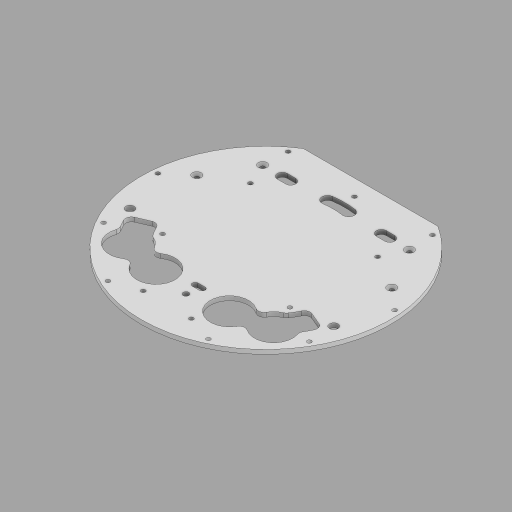
# Autodesk Inventor part: V_2
Saved by Autodesk Inventor 2024.2 (Build 282272000, 272)
## iProperties
Created: 2023-12-16
Part Number: V_2
Material: Типовые
Document SubType Name: Modeling
Designer: Фёдор
Density: 1 g/cm^3
Appearance: По умолчанию
Author: Фёдор
Autodesk Inventor part; units mm, degrees
ref_plane "YZ Plane" through (0, 0, 0) normal (1, 0, 0) x (0, 1, 0)
ref_plane "XZ Plane" through (0, 0, 0) normal (0, 1, 0) x (-1, 0, 0)
ref_plane "XY Plane" through (0, 0, 0) normal (0, 0, 1) x (1, 0, 0)
sketch "Эскиз1" plane through (0, 0, 0) normal (0, 1, 0) x (-1, 0, 0)
  arc A0 (110.5702, -95.2576) -> (50, 9.653) centre (25, -74.7211) ccw
  line L0 (102.2104, -90.4311) -> (110.5702, -95.2576) construction
  line L1 (102.2104, -90.4311) -> (77.2104, -133.7324) construction
  line L2 (85.5702, -138.5589) -> (77.2104, -133.7324) construction
  arc A1 (70, -150.3452) -> (85.5702, -138.5589) centre (25, -74.7211) ccw
  line L3 (-20, -150.3452) -> (70, -150.3452)
  arc A2 (-35.5702, -138.5589) -> (-20, -150.3452) centre (25, -74.7211) ccw
  line L4 (-27.2104, -133.7324) -> (-35.5702, -138.5589) construction
  line L5 (-27.2104, -133.7324) -> (-52.2104, -90.4311) construction
  line L6 (-60.5702, -95.2576) -> (-52.2104, -90.4311) construction
  arc A3 (0, 9.653) -> (-60.5702, -95.2576) centre (25, -74.7211) ccw
  line L7 (0, 0) -> (0, 9.653) construction
  line L8 (0, 0) -> (50, 0) construction
  line L9 (50, 9.653) -> (50, 0) construction
  line L10 (25, -74.7211) -> (25, 8.2789) construction
  line L11 (0, 0) -> (50, 0) construction
  line L12 (50, 0) -> (50, -10) construction
  line L13 (50, -10) -> (0, -10) construction
  line L14 (0, -10) -> (0, 0) construction
  line L15 (0, -5) -> (50, -5) construction
  circle A4 centre (8, -5) radius 1.5
  circle A5 centre (42, -5) radius 1.5
  circle A6 centre (93.8803, -94.8593) radius 1.5
  circle A7 centre (76.8803, -124.3042) radius 1.5
  circle A8 centre (-26.8803, -124.3042) radius 1.5
  circle A9 centre (-43.8803, -94.8593) radius 1.5
  circle A10 centre (25, -74.7211) radius 88
  point P0 (0, 0)
  point P1 (-35.5702, -138.5589)
  point P2 (85.5702, -138.5589)
  point P3 (110.5702, -95.2576)
  point P4 (50, 9.653)
  point P5 (0, 9.653)
  dimension "d25" = 50
  dimension "d26" = 10
  dimension "d27" = 3
  dimension "d28" = 3
  dimension "d29" = 8
  dimension "d30" = 8
  dimension "d33" = 360
  constraints: 32 end point, 10 centre point, 8 point on circle, 3 horizontal, 3 vertical, 2 coincident, 2 midpoint, 2 parallel, 2 point on line, 1 perpendicular, 45 other
  measures "d25" distance of L12.end L13.end
  measures "d26" distance of L11.end L12.end
  measures "d27" diameter of A4
  measures "d28" diameter of A5
  measures "d29" distance from line of L14 A4.centre
  measures "d30" distance from line of L12 A5.centre
extrude "Выдавливание1" add sketch "Эскиз1" along normal blind 3 contours A10 A1 L3 A2 A3 A0
sketch "Эскиз8" plane through (0, 3, 0) normal (0, 1, 0) x (1, 0, 0)
  circle A0 centre (-8, 5) radius 1.5 projected
  circle A1 centre (-42, 5) radius 1.5 projected
  circle A2 centre (-93.8803, 94.8593) radius 1.5 projected
  circle A3 centre (-76.8803, 124.3042) radius 1.5 projected
  circle A4 centre (26.8803, 124.3042) radius 1.5 projected
  circle A5 centre (43.8803, 94.8593) radius 1.5 projected
  arc A6 (-70, 150.3452) -> (20, 150.3452) centre (-25, 74.7211) ccw projected
  line L0 (-25, 74.7211) -> (-186.093, 74.7211) construction
  circle A7 centre (-25, 74.7211) radius 80
  line L1 (-25, 74.7211) -> (-112.6651, 82.3909) construction
  line L2 (-112.6651, 82.3909) -> (-108.6804, 82.0422) construction
  circle A8 centre (-108.6804, 82.0422) radius 1.5
  line L3 (-25, 74.7211) -> (-78.4735, 144.611) construction
  circle A9 centre (-76.0429, 141.4342) radius 1.5
  line L4 (-25, 74.7211) -> (-62.1904, -5.0339) construction
  line L5 (-25, 74.7211) -> (-101.2102, 30.7211) construction
  circle A10 centre (-60.4999, -1.4087) radius 1.5
  circle A11 centre (-97.7461, 32.7211) radius 1.5
  line L6 (-25, 74.7211) -> (-25, -13.2789) construction
  circle A12 centre (58.6804, 82.0422) radius 1.5
  circle A13 centre (26.0429, 141.4342) radius 1.5
  circle A14 centre (10.4999, -1.4087) radius 1.5
  circle A15 centre (47.7461, 32.7211) radius 1.5
  line L7 (-68, 140.8452) -> (18, 140.8452) projected
  line L8 (-25, 140.8452) -> (-25, 137.3452) construction
  circle A16 centre (-25, 137.3452) radius 1.5
  line L9 (20, 150.3452) -> (-70, 150.3452) projected
  point P0 (0, 0)
  dimension "d47" = 8
  dimension "d48" = 5
  dimension "d50" = 4
  dimension "d51" = 3
  dimension "d52" = 52.58
  dimension "d53" = 3
  dimension "d54" = 4
  dimension "d55" = 3
  dimension "d56" = 3
  dimension "d57" = 4
  dimension "d58" = 4
  dimension "d59" = 30
  dimension "d60" = 65
  dimension "d61" = 3.5
  dimension "d62" = 3
  constraints: 16 end point, 10 centre point, 5 point on circle, 4 point on line, 4 symmetric about line, 3 coincident, 2 horizontal, 1 midpoint, 1 vertical, 4 other
  measures "d47" radial gap between concentric circles of A6 A7
  measures "d48" angle of L1 L0
  measures "d50" distance of L1.end L2.end
  measures "d51" diameter of A8
  measures "d52" angle of L3 L0
  measures "d53" diameter of A9
  measures "d54" distance of L3.end A9.centre
  measures "d55" diameter of A10
  measures "d56" diameter of A11
  measures "d57" distance of L5.end A11.centre
  measures "d58" distance of L4.end A10.centre
  measures "d59" angle of L5 L0
  measures "d60" angle of L0 L4
  measures "d61" distance of L8.start L8.end
  measures "d62" diameter of A16
extrude "Выдавливание6" cut sketch "Эскиз8" against normal blind 10 contours A8 | A9 | A10 | A11 | A12 | A13 | A14 | A15 | A16
sketch "Эскиз10" plane through (0, 3, 0) normal (0, 1, 0) x (1, 0, 0)
  arc A0 (-70, 150.3452) -> (20, 150.3452) centre (-25, 74.7211) ccw projected
  line L0 (-72.591, 148.7421) -> (22.591, 148.7421)
  circle A1 centre (26.0429, 141.4342) radius 1.5 projected
  circle A2 centre (-60.4999, -1.4087) radius 1.5 projected
  circle A3 centre (-97.7461, 32.7211) radius 1.5 projected
  circle A4 centre (58.6804, 82.0422) radius 1.5 projected
  circle A5 centre (-25, 137.3452) radius 1.5 projected
  circle A6 centre (10.4999, -1.4087) radius 1.5 projected
  circle A7 centre (-108.6804, 82.0422) radius 1.5 projected
  circle A8 centre (47.7461, 32.7211) radius 1.5 projected
  circle A9 centre (-76.0429, 141.4342) radius 1.5 projected
  arc A10 (-70, 150.3452) -> (20, 150.3452) centre (-25, 74.7211) ccw projected
  line L1 (20, 150.3452) -> (-70, 150.3452) projected
  point P0 (0, 0)
  point P1 (20, 150.3452)
  dimension "d71" = 95.182
  constraints: 2 end point, 2 point on circle, 1 horizontal
  measures "d71" distance of L0.start L0.end
extrude "Выдавливание7" cut sketch "Эскиз10" against normal blind 10 contours L1 A0 L0
sketch "Эскиз11" plane through (0, 3, 0) normal (0, 1, 0) x (1, 0, 0)
  line L0 (22.591, 148.7421) -> (-72.591, 148.7421) projected
  arc A0 (-72.591, 148.7421) -> (22.591, 148.7421) centre (-25, 74.7211) ccw projected
  circle A1 centre (26.0429, 141.4342) radius 1.5 projected
  circle A2 centre (-60.4999, -1.4087) radius 1.5 projected
  circle A3 centre (-97.7461, 32.7211) radius 1.5 projected
  circle A4 centre (58.6804, 82.0422) radius 1.5 projected
  circle A5 centre (-25, 137.3452) radius 1.5 projected
  circle A6 centre (10.4999, -1.4087) radius 1.5 projected
  circle A7 centre (-108.6804, 82.0422) radius 1.5 projected
  circle A8 centre (47.7461, 32.7211) radius 1.5 projected
  circle A9 centre (-76.0429, 141.4342) radius 1.5 projected
  circle A10 centre (-25, 74.7211) radius 65
  line L1 (-74.6085, 116.7211) -> (24.6085, 116.7211)
  line L2 (22.591, 148.7421) -> (-72.591, 148.7421) projected
  line L3 (-80.3986, 108.7211) -> (30.3986, 108.7211) construction
  circle A11 centre (-70, 108.7211) radius 1.5
  circle A12 centre (20, 108.7211) radius 1.5
  circle A13 centre (-25, 74.7211) radius 56.5155 construction
  line L4 (-25, 74.7211) -> (-25, 9.7211) construction
  circle A14 centre (-25, 18.2056) radius 2
  line L5 (-74.0918, 46.7211) -> (24.0918, 46.7211) construction
  circle A15 centre (-70, 46.7211) radius 1.5
  circle A16 centre (20, 46.7211) radius 1.5
  point P0 (0, 0)
  dimension "d74" = 130
  dimension "d75" = 42
  dimension "d76" = 8
  dimension "d77" = 3
  dimension "d78" = 3
  dimension "d79" = 45
  dimension "d80" = 45
  dimension "d81" = 113.031
  dimension "d82" = 4
  dimension "d83" = 70
  dimension "d91" = 3
  dimension "d92" = 3
  dimension "d93" = 45
  dimension "d94" = 45
  dimension "d130" = 34
  dimension "d131" = 62
  dimension "d132" = 56.5155
  constraints: 8 end point, 8 point on circle, 7 centre point, 5 point on line, 3 horizontal, 2 coincident, 1 parallel, 1 vertical
  measures "d74" diameter of A10
  measures "d75" distance from line of L1 A0.centre
  measures "d76" distance between parallel lines of L1 L3
  measures "d77" diameter of A11
  measures "d78" diameter of A12
  measures "d79" horizontal distance of A11.centre A0.centre
  measures "d80" horizontal distance of A12.centre A0.centre
  measures "d81" diameter of A13
  measures "d82" diameter of A14
  measures "d83" distance between parallel lines of L1 L5
  measures "d91" diameter of A15
  measures "d92" diameter of A16
  measures "d93" horizontal distance of A0.centre A16.centre
  measures "d94" horizontal distance of A0.centre A15.centre
  measures "d130" distance from line of L3 A0.centre
  measures "d131" distance between parallel lines of L5 L3
  measures "d132" distance of A14.centre A0.centre
extrude "Выдавливание8" cut sketch "Эскиз11" against normal blind 10 contours A11 | A12 | A14 | A15 | A16
chamfer "Фаска3" [suppressed]
sketch "Эскиз12" plane through (0, 0, 0) normal (0, -1, 0) x (1, 0, 0)
  circle A0 centre (26.0429, -141.4342) radius 1.5 projected
  circle A1 centre (-60.4999, 1.4087) radius 1.5 projected
  circle A2 centre (-97.7461, -32.7211) radius 1.5 projected
  circle A3 centre (58.6804, -82.0422) radius 1.5 projected
  circle A4 centre (-25, -137.3452) radius 1.5 projected
  circle A5 centre (10.4999, 1.4087) radius 1.5 projected
  circle A6 centre (-108.6804, -82.0422) radius 1.5 projected
  circle A7 centre (47.7461, -32.7211) radius 1.5 projected
  circle A8 centre (-76.0429, -141.4342) radius 1.5 projected
  line L0 (-72.591, -148.7421) -> (22.591, -148.7421) projected
  arc A9 (22.591, -148.7421) -> (-72.591, -148.7421) centre (-25, -74.7211) ccw projected
  circle A10 centre (43.8803, -94.8593) radius 1.5 projected
  circle A11 centre (26.8803, -124.3042) radius 1.5 projected
  circle A12 centre (-76.8803, -124.3042) radius 1.5 projected
  circle A13 centre (-93.8803, -94.8593) radius 1.5 projected
  circle A14 centre (-42, -5) radius 1.5 projected
  circle A15 centre (-8, -5) radius 1.5 projected
  line L1 (59.664, -50.7211) -> (-109.664, -50.7211) construction
  circle A16 centre (47, -50.7211) radius 3
  circle A17 centre (-97, -50.7211) radius 3
  point P0 (0, 0)
  dimension "d95" = 24
  dimension "d96" = 6
  dimension "d97" = 72
  dimension "d98" = 6
  dimension "d99" = 72
  constraints: 2 centre point, 2 end point, 2 point on circle, 2 point on line, 1 horizontal
  measures "d95" distance from line of L1 A9.centre
  measures "d96" diameter of A16
  measures "d97" horizontal distance of A16.centre A9.centre
  measures "d98" diameter of A17
  measures "d99" horizontal distance of A17.centre A9.centre
extrude "Выдавливание9" cut sketch "Эскиз12" against normal blind 10 contours A16 | A17
sketch "Эскиз13" plane through (0, 3, 0) normal (0, 1, 0) x (1, 0, 0)
  circle A0 centre (-97, 50.7211) radius 3 projected
  circle A1 centre (47, 50.7211) radius 3 projected
  circle A2 centre (-70, 108.7211) radius 1.5 projected
  circle A3 centre (20, 108.7211) radius 1.5 projected
  circle A4 centre (20, 46.7211) radius 1.5 projected
  circle A5 centre (-25, 18.2056) radius 2 projected
  circle A6 centre (-70, 46.7211) radius 1.5 projected
  line L0 (22.591, 148.7421) -> (-72.591, 148.7421) projected
  arc A7 (-72.591, 148.7421) -> (22.591, 148.7421) centre (-25, 74.7211) ccw projected
  circle A8 centre (26.0429, 141.4342) radius 1.5 projected
  circle A9 centre (-60.4999, -1.4087) radius 1.5 projected
  circle A10 centre (-97.7461, 32.7211) radius 1.5 projected
  circle A11 centre (58.6804, 82.0422) radius 1.5 projected
  circle A12 centre (-25, 137.3452) radius 1.5 projected
  circle A13 centre (10.4999, -1.4087) radius 1.5 projected
  circle A14 centre (-108.6804, 82.0422) radius 1.5 projected
  circle A15 centre (47.7461, 32.7211) radius 1.5 projected
  circle A16 centre (-76.0429, 141.4342) radius 1.5 projected
  circle A17 centre (-25, 74.7211) radius 59
  line L1 (-25, 74.7211) -> (-25, 18.2056) construction
  arc A18 (-17.5, 125.7975) -> (-32.5, 125.7975) centre (-25, 74.7211) ccw construction
  arc A19 (-16.9189, 129.7551) -> (-33.0811, 129.7551) centre (-25, 74.7211) ccw
  arc A20 (-18.0811, 121.8399) -> (-31.9189, 121.8399) centre (-25, 74.7211) ccw
  arc A21 (-18.0811, 121.8399) -> (-16.9189, 129.7551) centre (-17.5, 125.7975) ccw
  arc A22 (-33.0811, 129.7551) -> (-31.9189, 121.8399) centre (-32.5, 125.7975) ccw
  line L2 (-25, 74.7211) -> (-25, 148.7421) construction
  circle A23 centre (-76.8803, 124.3042) radius 1.5 projected
  circle A24 centre (26.8803, 124.3042) radius 1.5 projected
  line L3 (-76.8803, 124.3042) -> (26.8803, 124.3042) construction
  line L4 (-57, 124.3042) -> (-63, 124.3042) construction
  line L5 (-57, 127.8042) -> (-63, 127.8042)
  line L6 (-63, 120.8042) -> (-57, 120.8042)
  arc A25 (-57, 120.8042) -> (-57, 127.8042) centre (-57, 124.3042) ccw
  arc A26 (-63, 127.8042) -> (-63, 120.8042) centre (-63, 124.3042) ccw
  line L7 (7, 124.3042) -> (13, 124.3042) construction
  line L8 (7, 127.8042) -> (13, 127.8042)
  line L9 (13, 120.8042) -> (7, 120.8042)
  arc A27 (7, 127.8042) -> (7, 120.8042) centre (7, 124.3042) ccw
  arc A28 (13, 120.8042) -> (13, 127.8042) centre (13, 124.3042) ccw
  point P0 (0, 0)
  point P1 (-25, 126.3452)
  point P2 (-20.7857, 133.5704)
  point P3 (-29.2143, 133.5704)
  point P4 (-60, 124.3042)
  point P5 (10, 124.3042)
  dimension "d102" = 118
  dimension "d106" = 4
  dimension "d107" = 15
  dimension "d110" = 11
  dimension "d140" = 7
  dimension "d141" = 3
  dimension "d142" = 35
  constraints: 22 end point, 19 point on circle, 10 centre point, 8 tangent, 7 symmetric about line, 3 coincident, 3 point on line, 2 midpoint, 1 horizontal, 1 parallel, 1 vertical, 2 other
  measures "d102" diameter of A17
  measures "d106" radius of A22
  measures "d107" distance of A18.start A18.end
  measures "d110" distance of A12.centre point (-25, 126.345)
  measures "d140" diameter of A26
  measures "d141" distance of point (-60, 124.304) L4.end
  measures "d142" horizontal distance of point (-25, 126.345) point (-60, 124.304)
extrude "Выдавливание10" cut sketch "Эскиз13" against normal blind 10 contours L9 A27 A17 | A17 A27 L8 A28 L9 | L6 A26 L5 A25 A17 | A17 A25 L6 | A21 A20 A22 A19
chamfer "Фаска4" distance 1.6 angle 45 4 edges at (-92.3803, 3, -94.8593) (-75.3803, 3, -124.3042) (28.3803, 3, -124.3042) (45.3803, 3, -94.8593)
sketch "Эскиз15" plane through (0, 3, 0) normal (0, 1, 0) x (1, 0, 0)
  circle A0 centre (26.8803, 124.3042) radius 3.1 projected
  circle A1 centre (-93.8803, 94.8593) radius 3.1 projected
  arc A2 (-33.0811, 129.7551) -> (-31.9189, 121.8399) centre (-32.5, 125.7975) ccw projected
  arc A3 (-16.9189, 129.7551) -> (-33.0811, 129.7551) centre (-25, 74.7211) ccw projected
  arc A4 (-18.0811, 121.8399) -> (-16.9189, 129.7551) centre (-17.5, 125.7975) ccw projected
  arc A5 (-18.0811, 121.8399) -> (-31.9189, 121.8399) centre (-25, 74.7211) ccw projected
  circle A6 centre (-97, 50.7211) radius 3 projected
  circle A7 centre (47, 50.7211) radius 3 projected
  circle A8 centre (-70, 108.7211) radius 1.5 projected
  circle A9 centre (20, 108.7211) radius 1.5 projected
  circle A10 centre (20, 46.7211) radius 1.5 projected
  circle A11 centre (-25, 18.2056) radius 2 projected
  circle A12 centre (-70, 46.7211) radius 1.5 projected
  line L0 (22.591, 148.7421) -> (-72.591, 148.7421) projected
  arc A13 (-72.591, 148.7421) -> (22.591, 148.7421) centre (-25, 74.7211) ccw projected
  circle A14 centre (26.0429, 141.4342) radius 1.5 projected
  circle A15 centre (-60.4999, -1.4087) radius 1.5 projected
  circle A16 centre (-97.7461, 32.7211) radius 1.5 projected
  circle A17 centre (58.6804, 82.0422) radius 1.5 projected
  circle A18 centre (-25, 137.3452) radius 1.5 projected
  circle A19 centre (10.4999, -1.4087) radius 1.5 projected
  circle A20 centre (-108.6804, 82.0422) radius 1.5 projected
  circle A21 centre (47.7461, 32.7211) radius 1.5 projected
  circle A22 centre (-76.0429, 141.4342) radius 1.5 projected
  circle A23 centre (-42, 5) radius 1.5 projected
  circle A24 centre (-8, 5) radius 1.5 projected
  circle A25 centre (-76.8803, 124.3042) radius 3.1 projected
  circle A26 centre (43.8803, 94.8593) radius 3.1 projected
  line L1 (-25, 74.7211) -> (-25, -13.2789) construction
  line L2 (-51, 23) -> (1, 23) construction
  line L3 (-51, 23) -> (-76.3336, 28.8487) construction
  line L4 (1, 23) -> (26.3336, 28.8487) construction
  circle A27 centre (-76.3336, 28.8487) radius 12.5 construction
  circle A28 centre (-51, 23) radius 12.5 construction
  circle A29 centre (1, 23) radius 12.5 construction
  circle A30 centre (26.3336, 28.8487) radius 12.5 construction
  circle A31 centre (-76.3336, 28.8487) radius 13.5
  circle A32 centre (-51, 23) radius 13.5
  circle A33 centre (26.3336, 28.8487) radius 13.5
  circle A34 centre (1, 23) radius 13.5
  point P0 (0, 0)
  point P1 (-25, 23)
  point P2 (14.4856, 22.3776)
  point P3 (-64.4856, 22.3776)
  dimension "d115" = 52
  dimension "d116" = 18
  dimension "d117" = 26
  dimension "d118" = 26
  dimension "d119" = 167
  dimension "d120" = 167
  dimension "d121" = 25
  dimension "d122" = 25
  dimension "d123" = 25
  dimension "d124" = 25
  dimension "d125" = 27
  dimension "d126" = 27
  constraints: 8 centre point, 8 end point, 6 coincident, 2 symmetric about line, 1 horizontal, 1 midpoint, 1 point on circle, 1 point on line, 2 other
  measures "d115" distance of L2.start L2.end
  measures "d116" distance from line of L2 A23.centre
  measures "d117" distance of L2.start L3.end
  measures "d118" distance of L2.end L4.end
  measures "d119" angle of L2 L3
  measures "d120" angle of L4 L2
  measures "d121" diameter of A27
  measures "d122" diameter of A28
  measures "d123" diameter of A29
  measures "d124" diameter of A30
  measures "d125" diameter of A31
  measures "d126" diameter of A32
extrude "Выдавливание11" cut sketch "Эскиз15" against normal through all contours A31 A32 | A31 A32 | A32 A31 | A33 A34 | A34 A33 | A33 A34
fillet "Сопряжение4" radius 4 4 edges at (-64.4856, 1.5, -22.3776) (-62.848, 1.5, -29.4711) (14.4856, 1.5, -22.3776) (12.848, 1.5, -29.4711)
sketch "Эскиз16" plane through (0, 3, 0) normal (0, 1, 0) x (1, 0, 0)
  arc A0 (-62.8046, 16.45) -> (-68.5951, 17.7868) centre (-66.3022, 14.5093) ccw projected
  arc A1 (-64.5291, 35.3987) -> (-68.5951, 17.7868) centre (-76.3336, 28.8487) ccw projected
  arc A2 (-64.5291, 35.3987) -> (-58.7385, 34.0619) centre (-61.0314, 37.3395) ccw projected
  arc A3 (-62.8046, 16.45) -> (-58.7385, 34.0619) centre (-51, 23) ccw projected
  arc A4 (18.5951, 17.7868) -> (12.8046, 16.45) centre (16.3022, 14.5093) ccw projected
  arc A5 (8.7385, 34.0619) -> (12.8046, 16.45) centre (1, 23) ccw projected
  arc A6 (8.7385, 34.0619) -> (14.5291, 35.3987) centre (11.0314, 37.3395) ccw projected
  arc A7 (18.5951, 17.7868) -> (14.5291, 35.3987) centre (26.3336, 28.8487) ccw projected
  circle A8 centre (26.8803, 124.3042) radius 3.1 projected
  circle A9 centre (-93.8803, 94.8593) radius 3.1 projected
  arc A10 (-33.0811, 129.7551) -> (-31.9189, 121.8399) centre (-32.5, 125.7975) ccw projected
  arc A11 (-16.9189, 129.7551) -> (-33.0811, 129.7551) centre (-25, 74.7211) ccw projected
  arc A12 (-18.0811, 121.8399) -> (-16.9189, 129.7551) centre (-17.5, 125.7975) ccw projected
  arc A13 (-18.0811, 121.8399) -> (-31.9189, 121.8399) centre (-25, 74.7211) ccw projected
  circle A14 centre (-97, 50.7211) radius 3 projected
  circle A15 centre (47, 50.7211) radius 3 projected
  circle A16 centre (-70, 108.7211) radius 1.5 projected
  circle A17 centre (20, 108.7211) radius 1.5 projected
  circle A18 centre (20, 46.7211) radius 1.5 projected
  circle A19 centre (-25, 18.2056) radius 2 projected
  circle A20 centre (-70, 46.7211) radius 1.5 projected
  line L0 (22.591, 148.7421) -> (-72.591, 148.7421) projected
  arc A21 (-72.591, 148.7421) -> (22.591, 148.7421) centre (-25, 74.7211) ccw projected
  circle A22 centre (26.0429, 141.4342) radius 1.5 projected
  circle A23 centre (-60.4999, -1.4087) radius 1.5 projected
  circle A24 centre (-97.7461, 32.7211) radius 1.5 projected
  circle A25 centre (58.6804, 82.0422) radius 1.5 projected
  circle A26 centre (-25, 137.3452) radius 1.5 projected
  circle A27 centre (10.4999, -1.4087) radius 1.5 projected
  circle A28 centre (-108.6804, 82.0422) radius 1.5 projected
  circle A29 centre (47.7461, 32.7211) radius 1.5 projected
  circle A30 centre (-76.0429, 141.4342) radius 1.5 projected
  circle A31 centre (-42, 5) radius 1.5 projected
  circle A32 centre (-8, 5) radius 1.5 projected
  circle A33 centre (-76.8803, 124.3042) radius 3.1 projected
  circle A34 centre (43.8803, 94.8593) radius 3.1 projected
  circle A35 centre (-25, 74.7211) radius 75
  circle A36 centre (-25, 74.7211) radius 57.5
  line L1 (-25, 74.7211) -> (-25, -13.2789) construction
  circle A37 centre (-25, 74.7211) radius 70 construction
  line L2 (-94.0379, 45.4163) -> (-77.929, 52.2541)
  line L3 (44.0379, 45.4163) -> (27.929, 52.2541)
  line L4 (-22.5, 27.2056) -> (-27.5, 27.2056) construction
  line L5 (-22.5, 29.2056) -> (-27.5, 29.2056)
  line L6 (-27.5, 25.2056) -> (-22.5, 25.2056)
  arc A38 (-22.5, 25.2056) -> (-22.5, 29.2056) centre (-22.5, 27.2056) ccw
  arc A39 (-27.5, 29.2056) -> (-27.5, 25.2056) centre (-27.5, 27.2056) ccw
  point P0 (0, 0)
  point P1 (27.929, 52.2541)
  point P2 (22.035, 41.6461)
  point P3 (38.4692, 34.7629)
  point P4 (-88.4692, 34.7629)
  point P5 (-72.035, 41.6461)
  point P6 (-25, 27.2056)
  dimension "d133" = 150
  dimension "d134" = 115
  dimension "d135" = 140
  dimension "d136" = 67
  dimension "d144" = 5
  dimension "d145" = 2
  dimension "d146" = 9
  constraints: 14 end point, 5 point on circle, 4 tangent, 3 centre point, 3 coincident, 2 symmetric about line, 1 line through centre, 1 midpoint, 1 parallel, 1 perpendicular, 1 point on line, 6 other
  measures "d135" diameter of A37
  measures "d136" angle of L1 L2
  measures "d144" distance of L4.start L4.end
  measures "d145" radius of A39
  measures "d146" distance of point (-25, 27.206) A19.centre
extrude "Выдавливание12" cut sketch "Эскиз16" against normal blind 10 contours A1 A35 L2 A36 | A7 A36 L3 A35 | A38 L6 A39 L5
fillet "Сопряжение5" radius 4 8 edges at (-94.0379, 1.5, -45.4163) (-77.929, 1.5, -52.2541) (-72.035, 1.5, -41.6461) (-88.4692, 1.5, -34.7629) (27.929, 1.5, -52.2541) (22.035, 1.5, -41.6461) (38.4692, 1.5, -34.7629) (44.0379, 1.5, -45.4163)
equation "\"d97\" = d99"
